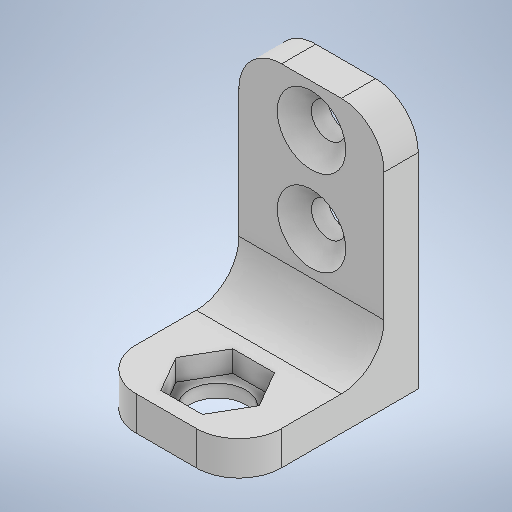
# Autodesk Inventor part: AntennaWallMount
Saved by Autodesk Inventor 2025.3 (Build 293356000, 356)
## iProperties
Created: 2025-07-17
Part Number: AntennaWallMount
Material: Generic
Document SubType Name: Modeling
Designer: vncnt
Density: 1 g/cm^3
Appearance: Default
Author: vncnt
Autodesk Inventor part; units mm, degrees
ref_plane "YZ Plane" through (0, 0, 0) normal (1, 0, 0) x (0, 1, 0)
ref_plane "XZ Plane" through (0, 0, 0) normal (0, 1, 0) x (-1, 0, 0)
ref_plane "XY Plane" through (0, 0, 0) normal (0, 0, 1) x (1, 0, 0)
sketch "Sketch1" plane through (0, 0, 0) normal (1, 0, 0) x (0, 1, 0)
  line L0 (0, 0) -> (25, 0)
  line L1 (25, 0) -> (25, -4)
  line L2 (25, -4) -> (0, -4)
  line L3 (0, -4) -> (0, 0)
  line L4 (0, 0) -> (-4, 0)
  line L5 (-4, 0) -> (-4, 17)
  line L6 (-4, 17) -> (0, 17)
  line L7 (0, 17) -> (0, 0)
  line L8 (0, 0) -> (-4, 0)
  line L9 (-4, 0) -> (-4, -4)
  line L10 (-4, -4) -> (0, -4)
  line L11 (0, -4) -> (0, 0)
  dimension "d0" = 25
  dimension "d1" = 4
  dimension "d2" = 4
  dimension "d3" = 17
  constraints: 24 end point, 6 parallel, 3 horizontal, 3 perpendicular
  measures "d0" distance of L1.end L2.end
  measures "d1" distance of L0.end L1.end
  measures "d2" distance of L5.end L6.end
  measures "d3" distance of L4.end L5.end
extrude "Extrusion1" add sketch "Sketch1" along normal blind 17
fillet "Fillet1" radius 5 1 edges at (8.5, 0, 0)
sketch "Sketch2" plane through (0, 0, 17) normal (0, 1, 0) x (1, 0, 0)
  line L0 (0, 0) -> (0, 21) projected
  line L1 (0, 12) -> (17, 12) projected
  line L2 (0, 0) -> (17, 12)
  line L3 (17, 0) -> (17, 21) projected
  line L4 (0, 12) -> (17, 0)
  line L5 (3.6214, 6) -> (6.0607, 10.225)
  line L6 (6.0607, 10.225) -> (10.9393, 10.225)
  line L7 (10.9393, 10.225) -> (13.3786, 6)
  line L8 (13.3786, 6) -> (10.9393, 1.775)
  line L9 (10.9393, 1.775) -> (6.0607, 1.775)
  line L10 (6.0607, 1.775) -> (3.6214, 6)
  point P0 (0, 17)
  point P1 (8.5, 6)
  dimension "d7" = 8.45
  constraints: 16 end point, 1 midpoint, 13 other
  measures "d7" distance between parallel lines of L8 L5
extrude "Extrusion2" cut sketch "Sketch2" against normal blind 2.5 contours L10 L5 L4 L2 | L2 L4 L8 L9 L10 | L5 L6 L7 L2 L4 | L2 L7 L8 L4
sketch "Sketch3" plane through (0, -2.5, 17) normal (0, 1, 0) x (1, 0, 0)
  line L0 (10.9393, 1.775) -> (6.0607, 1.775) projected
  line L1 (6.0607, 10.225) -> (10.9393, 1.775)
  line L2 (10.9393, 10.225) -> (13.3786, 6) projected
  line L3 (6.0607, 1.775) -> (10.9393, 10.225)
  circle A0 centre (8.5, 6) radius 3.3
  point P0 (0, 17)
  dimension "d10" = 6.6
  constraints: 4 end point, 1 centre point, 1 midpoint
  measures "d10" diameter of A0
extrude "Extrusion3" cut sketch "Sketch3" against normal through all contours A0 L3 L1 | L1 L3 A0 | A0 L1 L3 | L1 A0 L3
sketch "Sketch4" plane through (0, 25, 0) normal (0, 0, 1) x (1, 0, 0)
  line L0 (17, -20) -> (0, -20) projected
  line L1 (17, -29) -> (17, 0) projected
  line L2 (17, -20) -> (17, 0)
  line L3 (17, -10) -> (0, -10)
  line L4 (0, -29) -> (0, 0) projected
  line L5 (0, -20) -> (17, -10)
  line L6 (0, 0) -> (17, 0) projected
  line L7 (17, -10) -> (0, 0)
  line L8 (0, -10) -> (17, -20)
  line L9 (17, 0) -> (0, -10)
  circle A0 centre (8.5, -5) radius 2
  circle A1 centre (8.5, -15) radius 2
  point P0 (0, -25)
  dimension "d13" = 4
  dimension "d14" = 4
  constraints: 12 end point, 3 midpoint, 2 centre point, 1 horizontal, 1 point on line, 1 vertical
  measures "d13" diameter of A0
  measures "d14" diameter of A1
extrude "Extrusion4" cut sketch "Sketch4" against normal through all contours A1 L5 L8 | L8 L5 A1 | A1 L8 L5 | L5 L8 A1 | A0 L9 L7 | L7 L9 A0 | A0 L7 L9 | L9 L7 A0
chamfer "Chamfer1" distance 2 angle 45 2 edges at (6.5, 20, 0) (6.5, 10, 0)
fillet "Fillet2" radius 5 4 edges at (17, 25, -2) (0, 25, -2) (17, -2, 17) (0, -2, 17)
body "Solid1"
